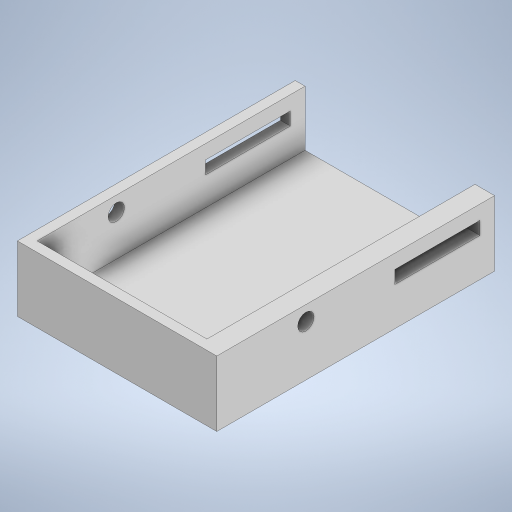
# Autodesk Inventor part: breadboard box v03
Saved by Autodesk Inventor 2023 (Build 270158000, 158)
## iProperties
Created: 2024-07-12
Part Number: breadboard box v03
Material: Generic
Document SubType Name: Modeling
Designer: Akramilab
Density: 1 g/cm^3
Appearance: Default
Author: Akramilab
Autodesk Inventor part; units mm, degrees
ref_plane "YZ Plane" through (0, 0, 0) normal (1, 0, 0) x (0, 1, 0)
ref_plane "XZ Plane" through (0, 0, 0) normal (0, 1, 0) x (-1, 0, 0)
ref_plane "XY Plane" through (0, 0, 0) normal (0, 0, 1) x (1, 0, 0)
sketch "Sketch2" plane through (0, 0, 0) normal (0, 1, 0) x (-1, 0, 0)
  line L0 (0, 0) -> (-58, 0)
  line L1 (-58, 0) -> (-58, 85)
  line L2 (-58, 85) -> (0, 85)
  line L3 (0, 85) -> (0, 0)
  dimension "d0" = 58
  dimension "d1" = 85
  constraints: 8 end point, 2 parallel, 1 horizontal, 1 perpendicular
  measures "d0" distance of L0.start L0.end
  measures "d1" distance between parallel lines of L2 L0
extrude "Extrusion1" add sketch "Sketch2" along normal blind 20
shell "Shell1" thickness 3 removed faces 1 at (19.3333, 20, 28.3333)
sketch "Sketch4" plane through (58, 0, 0) normal (0, 0, -1) x (-1, 0, 0)
  point P0 (58, 0)
sketch "Sketch5" plane through (3, 3, 3) normal (0, 0, 1) x (1, 0, 0)
  line L0 (0, 0) -> (0, 17) projected
  line L1 (0, 17) -> (52, 17) projected
  line L2 (0, 0) -> (52, 0)
  line L3 (52, 0) -> (52, 17)
  line L4 (52, 17) -> (0, 17)
  line L5 (0, 17) -> (0, 0)
  point P0 (-3, -3)
  constraints: 8 end point, 2 parallel, 1 horizontal, 1 perpendicular
extrude "Extrusion3" cut sketch "Sketch5" against normal blind 10
sketch "Sketch6" plane through (0, 0, 0) normal (-1, 0, 0) x (0, 0, 1)
  line L0 (4.5, 15.7) -> (30.5, 15.7)
  line L1 (30.5, 15.7) -> (30.5, 11.7)
  line L2 (30.5, 11.7) -> (4.5, 11.7)
  line L3 (4.5, 11.7) -> (4.5, 15.7)
  line L4 (0, 0) -> (0, 20) projected
  line L5 (0, 0) -> (85, 0) projected
  line L6 (0, 20) -> (85, 20) projected
  dimension "d19" = 26
  dimension "d20" = 4
  dimension "d21" = 4.5
  dimension "d34" = 11.7
  constraints: 8 end point, 2 parallel, 1 horizontal, 1 perpendicular
  measures "d19" distance of L0.start L0.end
  measures "d20" distance of L2.end L0.start
  measures "d21" distance between parallel lines of L4 L3
  measures "d34" distance between parallel lines of L2 L5
sketch "Sketch7" plane through (58, 0, 85) normal (1, 0, 0) x (0, 0, -1)
  line L0 (0, 0) -> (85, 0) projected
  line L1 (0, 20) -> (85, 20)
  line L2 (85, 20) -> (85, 0)
  line L3 (85, 0) -> (0, 0)
  line L4 (0, 0) -> (0, 20)
  constraints: 8 end point, 2 parallel, 1 horizontal, 1 perpendicular
extrude "Extrusion5" add sketch "Sketch7" along normal blind 3
extrude "Extrusion6" cut sketch "Sketch6" against normal through all
sketch "Sketch8" plane through (0, 0, 0) normal (-1, 0, 0) x (0, 0, 1)
  circle A0 centre (57.75, 15.5) radius 2.5
  line L0 (0, 20) -> (85, 20) projected
  line L1 (85, 0) -> (85, 20) projected
  line L2 (30.5, 15.7) -> (30.5, 11.7) projected
  point P0 (0, 0)
  point P1 (30.5, 13.7)
  dimension "d29" = 5
  dimension "d32" = 4.5
  dimension "d35" = 54.5
  dimension "d36" = 27.25
  constraints: 1 centre point, 1 coincident, 1 midpoint
  measures "d29" diameter of A0
  measures "d32" distance from line of L0 A0.centre
  measures "d35" distance from line of L1 point (30.5, 13.7)
  measures "d36" distance from line of L1 A0.centre
extrude "Extrusion7" cut sketch "Sketch8" against normal through all
equation "\"d36\" = 0.5 * d35"
body "Solid1"
